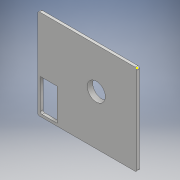
# Autodesk Inventor part: StaniceBoxTop
Saved by Autodesk Inventor 2017 (Build 210142000, 142)
## iProperties
Created: 2019-01-30
Part Number: StaniceBoxTop
Material: Generic
Document SubType Name: Modeling
Designer: Denis Kurka
Density: 1 g/cm^3
Appearance: Default
Author: Denis Kurka
Autodesk Inventor part; units mm, degrees
ref_plane "YZ Plane" through (0, 0, 0) normal (1, 0, 0) x (0, 1, 0)
ref_plane "XZ Plane" through (0, 0, 0) normal (0, 1, 0) x (-1, 0, 0)
ref_plane "XY Plane" through (0, 0, 0) normal (0, 0, 1) x (1, 0, 0)
sketch "Sketch1" plane through (0, 0, 0) normal (0, 1, 0) x (-1, 0, 0)
  line L0 (0, 0) -> (110, 0)
  line L1 (110, 0) -> (110, -100)
  line L2 (110, -100) -> (0, -100)
  line L3 (0, -100) -> (0, 0)
  dimension "d0" = 100
  dimension "d1" = 110
  constraints: 8 end point, 2 parallel, 1 horizontal, 1 perpendicular
  measures "d0" distance of L0.end L1.end
  measures "d1" distance of L1.end L2.end
extrude "Extrusion1" add sketch "Sketch1" along normal blind 3
sketch "Sketch2" plane through (0, 3, 0) normal (0, 1, 0) x (1, 0, 0)
  line L0 (-106.5, 3.5) -> (-3.5, 3.5)
  line L1 (-3.5, 3.5) -> (-3.5, 96.5)
  line L2 (-3.5, 96.5) -> (-106.5, 96.5)
  line L3 (-106.5, 96.5) -> (-106.5, 3.5)
  line L4 (-110, 100) -> (-110, 0) projected
  line L5 (-110, 0) -> (0, 0) projected
  line L6 (0, 100) -> (-110, 100) projected
  line L7 (0, 0) -> (0, 100) projected
  dimension "d4" = 3.5
  dimension "d5" = 3.5
  dimension "d6" = 3.5
  dimension "d7" = 3.5
  constraints: 8 end point, 2 parallel, 1 horizontal, 1 perpendicular
  measures "d4" distance between parallel lines of L4 L3
  measures "d5" distance between parallel lines of L5 L0
  measures "d6" distance between parallel lines of L6 L2
  measures "d7" distance between parallel lines of L7 L1
extrude "Extrusion2" add sketch "Sketch2" along normal blind 3 contours L3 L2 L1 L0
fillet "Fillet1" radius 2 8 edges at (0, 1.5, 0) (-3.5, 4.5, -3.5) (-110, 1.5, 0) (-106.5, 4.5, -3.5) (-106.5, 4.5, -96.5) (-110, 1.5, -100) (-3.5, 4.5, -96.5) (0, 1.5, -100)
sketch "Sketch3" plane through (0, 0, 0) normal (0, -1, 0) x (1, 0, 0)
  line L0 (-107, -97) -> (-88.5, -97)
  line L1 (-88.5, -97) -> (-88.5, -61.5)
  line L2 (-88.5, -61.5) -> (-107, -61.5)
  line L3 (-107, -61.5) -> (-107, -97)
  line L4 (-108, -100) -> (-2, -100) projected
  line L5 (-110, -2) -> (-110, -98) projected
  point P0 (0, 0)
  dimension "d11" = 35.5
  dimension "d12" = 18.5
  dimension "d13" = 3
  dimension "d14" = 3
  constraints: 8 end point, 2 parallel, 1 horizontal, 1 perpendicular
  measures "d11" distance of L0.end L1.end
  measures "d12" distance of L1.end L2.end
  measures "d13" distance between parallel lines of L4 L0
  measures "d14" distance between parallel lines of L5 L3
extrude "Extrusion3" cut sketch "Sketch3" against normal blind 10
fillet "Fillet2" radius 2 1 edges at (-107, 1.5, -97)
sketch "Sketch4" plane through (0, 0, 0) normal (0, -1, 0) x (1, 0, 0)
  circle A0 centre (-45, -45) radius 10
  line L0 (0, -98) -> (0, -2) projected
  line L1 (-2, 0) -> (-108, 0) projected
  point P0 (0, 0)
  dimension "d18" = 20
  dimension "d20" = 45
  dimension "d21" = 45
  constraints: 1 centre point
  measures "d18" diameter of A0
  measures "d20" distance from line of A0.centre L0
  measures "d21" distance from line of A0.centre L1
extrude "Extrusion4" cut sketch "Sketch4" against normal blind 10
sketch "Sketch5" plane through (0, 0, 0) normal (0, -1, 0) x (1, 0, 0)
  point P0 (0, 0)
body "Solid1"
